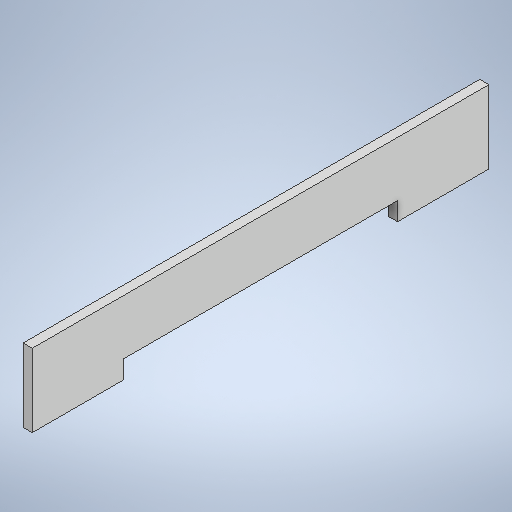
# Autodesk Inventor part: cover
Saved by Autodesk Inventor 2025.3 (Build 293356030, 356C)
## iProperties
Created: 2026-06-26
Part Number: cover
Material: Generic
Document SubType Name: Modeling
Designer: user
Density: 1 g/cm^3
Appearance: Default
Author: user
Autodesk Inventor part; units mm, degrees
ref_plane "YZ Plane" through (0, 0, 0) normal (1, 0, 0) x (0, 1, 0)
ref_plane "XZ Plane" through (0, 0, 0) normal (0, 1, 0) x (-1, 0, 0)
ref_plane "XY Plane" through (0, 0, 0) normal (0, 0, 1) x (1, 0, 0)
sketch "Sketch1" plane through (0, 0, 0) normal (1, 0, 0) x (0, 1, 0)
  line L0 (0, 0) -> (40, 0)
  line L1 (40, 0) -> (40, -50)
  line L2 (0, 0) -> (10, 0)
  line L3 (10, -50) -> (0, -50)
  line L4 (0, -50) -> (0, 0)
  line L5 (40, -50) -> (40, -250)
  line L6 (40, -250) -> (0, -250)
  line L7 (0, -250) -> (0, -200)
  line L8 (0, -200) -> (10, -200)
  line L9 (10, -200) -> (10, -50)
  dimension "d0" = 40
  dimension "d4" = 50
  dimension "d5" = 10
  dimension "d8" = 250
  dimension "d9" = 50
  constraints: 20 end point, 5 perpendicular, 2 horizontal, 1 parallel, 1 vertical
  measures "d0" distance of L0.start L0.end
  measures "d4" distance of L6.end L7.end
  measures "d5" distance of L7.end L8.end
  measures "d8" distance between parallel lines of L0 L6
  measures "d9" distance of L3.end L0.start
extrude "Extrusion1" add sketch "Sketch1" along normal blind 5
body "Solid1"
